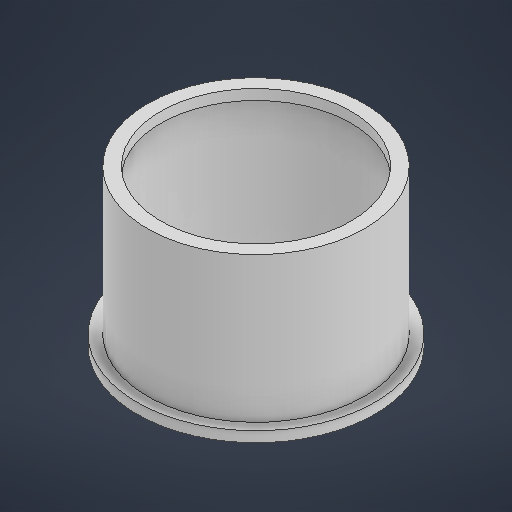
# Autodesk Inventor part: Cylinder  Segment - 10
Saved by Autodesk Inventor 2025 (Build 290162000, 162)
## iProperties
Created: 2024-04-11
Part Number: Cylinder  Segment - 10
Material: Generic
Document SubType Name: Modeling
Designer: Thienan Hoang
Density: 1 g/cm^3
Appearance: Default
Author: Thienan Hoang
Autodesk Inventor part; units mm, degrees
ref_plane "YZ Plane" through (0, 0, 0) normal (1, 0, 0) x (0, 1, 0)
ref_plane "XZ Plane" through (0, 0, 0) normal (0, 1, 0) x (-1, 0, 0)
sketch "Sketch1" plane through (0, 0, 0) normal (0, 1, 0) x (-1, 0, 0)
  circle A0 centre (0, 0) radius 57.25
  circle A1 centre (0, 0) radius 52.25
  circle A2 centre (0, 0) radius 50.4125
  circle A3 centre (0, 0) radius 9.5
  dimension "Absolute_Diameter" = 114.5
  dimension "Diameter_No_Outer_Lip" = 104.5
  dimension "Inner_Cylinder_Diameter" = 100.825
  dimension "Lip_Diameter" = 19
  constraints: 4 centre point, 4 coincident
  measures "Absolute_Diameter" diameter of A0
  measures "Diameter_No_Outer_Lip" diameter of A1
  measures "Inner_Cylinder_Diameter" diameter of A2
  measures "Lip_Diameter" diameter of A3
extrude "Extrusion1" add sketch "Sketch1" along normal blind 5 contours A0
extrude "Extrusion2" add sketch "Sketch1" along normal blind 75 contours A1
sketch "Sketch2" plane through (0, 75, 0) normal (0, 1, 0) x (1, 0, 0)
  circle A0 centre (0, 0) radius 52.25
  circle A1 centre (0, 0) radius 45.875
  dimension "Lip_Diameter_Out" = 104.5
  dimension "Inner_Lip_Diameter" = 91.75
  constraints: 2 centre point, 1 coincident
  measures "Lip_Diameter_Out" diameter of A0
  measures "Inner_Lip_Diameter" diameter of A1
extrude "Extrusion7" add sketch "Sketch2" against normal blind 5
ref_plane "Work Plane2" through (0, 10, 0) normal (0, 1, 0) x (1, 0, 0)
sketch "Sketch3" plane through (0, 10, 0) normal (0, 1, 0) x (1, 0, 0)
  circle A0 centre (0, 0) radius 127.5
  circle A1 centre (0, 127.5) radius 2.75
  circle A2 centre (-74.9426, 103.1497) radius 2.75
  circle A3 centre (-121.2597, 39.3997) radius 2.75
  circle A4 centre (-121.2597, -39.3997) radius 2.75
  circle A5 centre (-74.9426, -103.1497) radius 2.75
  circle A6 centre (0, -127.5) radius 2.75
  circle A7 centre (74.9426, -103.1497) radius 2.75
  circle A8 centre (121.2597, -39.3997) radius 2.75
  circle A9 centre (121.2597, 39.3997) radius 2.75
  circle A10 centre (74.9426, 103.1497) radius 2.75
  dimension "d27" = 255
  dimension "d229" = 5.5
  dimension "d232" = 360
  constraints: 10 centre point, 1 coincident, 1 vertical alignment, 23 other
  measures "d229" diameter of A1
extrude "Extrusion8" [suppressed]
sketch "Sketch24" plane through (0, 0, 0) normal (0, -1, 0) x (1, 0, 0)
  circle A0 centre (0, 0) radius 112.0375
  arc A1 (-85.157, -104.7535) -> (32.5, -131.0296) centre (0, 0) ccw
  circle A2 centre (0, 0) radius 133
  line L0 (-32.5, -70.125) -> (32.5, -70.125)
  line L1 (32.5, -70.125) -> (32.5, -160.125)
  line L2 (32.5, -160.125) -> (-32.5, -160.125)
  line L3 (-32.5, -160.125) -> (-32.5, -70.125)
  line L4 (-31, -158.625) -> (31, -158.625)
  line L5 (31, -158.625) -> (31, -71.625)
  line L6 (31, -71.625) -> (-31, -71.625)
  line L7 (-31, -71.625) -> (-31, -158.625)
  line L8 (-85.157, -65.125) -> (-46.3, -65.125)
  line L9 (-46.3, -65.125) -> (-46.3, -151.2985)
  line L10 (-46.3, -151.2985) -> (-85.157, -151.2985)
  line L11 (-85.157, -151.2985) -> (-85.157, -65.125)
  arc A3 (32.5, -131.0296) -> (-85.157, -104.7535) centre (0, 0) ccw
  line L12 (0, -71.625) -> (0, -158.625)
  line L13 (-83.157, -149.2985) -> (-48.3, -149.2985)
  line L14 (-48.3, -149.2985) -> (-48.3, -67.125)
  line L15 (-48.3, -67.125) -> (-83.157, -67.125)
  line L16 (-83.157, -67.125) -> (-83.157, -149.2985)
  line L17 (85.157, -65.125) -> (46.3, -65.125)
  line L18 (46.3, -65.125) -> (46.3, -151.2985)
  line L19 (46.3, -151.2985) -> (85.157, -151.2985)
  line L20 (85.157, -151.2985) -> (85.157, -65.125)
  line L21 (83.157, -149.2985) -> (48.3, -149.2985)
  line L22 (48.3, -149.2985) -> (48.3, -67.125)
  line L23 (48.3, -67.125) -> (83.157, -67.125)
  line L24 (83.157, -67.125) -> (83.157, -149.2985)
  circle A4 centre (0, 0) radius 120
  point P0 (0, -135)
  point P1 (48.3, -126.0639)
  point P2 (83.157, -106.3481)
  point P3 (-31, -131.3925)
  point P4 (31, -131.3925)
  point P5 (-83.157, -106.3481)
  point P6 (-48.3, -126.0639)
  point P7 (46.3, -126.8121)
  point P8 (85.157, -104.7535)
  point P9 (-32.5, -131.0296)
  point P10 (-46.3, -126.8121)
  point P11 (48.3, -109.8504)
  point P12 (48.3, -101.0916)
  point P13 (31, -107.6634)
  point P14 (31, -115.9267)
  point P15 (-48.3, -109.8504)
  point P16 (-31, -115.9267)
  point P17 (-31, -107.6634)
  point P18 (-48.3, -101.0916)
  dimension "d234" = 2
  dimension "d235" = 65
  dimension "d237" = 1.5
  dimension "d238" = 11.113
  dimension "d240" = 20.9625
  dimension "d241" = 270
  dimension "d242" = 90
  dimension "d243" = 153.238
  dimension "d244" = 228.338
  dimension "d247" = 2
  dimension "d248" = 129.75
  dimension "d253" = 240
  constraints: 50 end point, 8 parallel, 8 symmetric about line, 5 centre point, 5 point on circle, 4 perpendicular, 3 coincident, 2 horizontal, 2 midpoint, 2 point on line, 6 other
  measures "d234" radial gap between concentric circles of A1 A2
  measures "d235" distance of L1.end L2.end
  measures "d237" distance between parallel lines of L2 L4
  measures "d240" radial gap between concentric circles of A2 A0
  measures "d241" diameter of A1
  measures "d247" distance between parallel lines of L10 L13
  measures "d253" diameter of A4
extrude "Extrusion30" [suppressed]
extrude "Extrusion31" [suppressed]
extrude "Extrusion32" [suppressed]
fillet "Fillet14" [suppressed]
fillet "Fillet15" [suppressed]
fillet "Fillet16" [suppressed]
fillet "Fillet17" [suppressed]
fillet "Fillet18" [suppressed]
sketch "Sketch25" plane through (0, 70, 0) normal (0, -1, 0) x (1, 0, 0)
  circle A0 centre (0, 0) radius 112.0375
  circle A1 centre (0, 0) radius 115
  constraints: 2 centre point, 2 coincident
extrude "Extrusion33" [suppressed]
body "Solid1"
